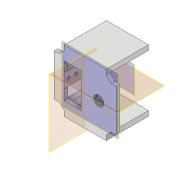
# Autodesk Inventor part: 30_Cube_Z_Focus_MGN_NEMA_base_v3
Saved by Autodesk Inventor 2022 (Build 260153000, 153)
## iProperties
Created: 2021-04-25
Part Number: 30_Cube_Z_Focus_MGN_NEMA_base_v3
Material: Generic
Document SubType Name: Modeling
Designer: diederichbenedict
Density: 1 g/cm^3
Appearance: Smooth - White
Author: diederichbenedict
Autodesk Inventor part; units mm, degrees
ref_plane "Work Plane1" through (0, 0, 6.7734) normal (0, 0, -1) x (-1, 0, 0)
sketch "Sketch1" plane through (0, 0, 6.7734) normal (0, 0, -1) x (-1, 0, 0)
  arc A0 (24.85, 22.85) -> (22.85, 24.85) centre (22.85, 22.85) ccw construction
  line L0 (22.85, 24.85) -> (-16.97, 24.85) construction
  line L1 (-16.97, 24.85) -> (-16.97, 21.15) construction
  line L2 (-16.97, 21.15) -> (16.97, 21.15) construction
  line L3 (16.97, 16.97) -> (16.97, 21.15) construction
  line L4 (21.15, 16.97) -> (16.97, 16.97) construction
  line L5 (21.15, 16.97) -> (21.15, -16.97) construction
  line L6 (21.15, -16.97) -> (24.85, -16.97) construction
  line L7 (24.85, -16.97) -> (24.85, 22.85) construction
  line L8 (23.75, 23.25) -> (23.75, 18.15) construction
  arc A1 (23.25, 17.65) -> (23.75, 18.15) centre (23.25, 18.15) ccw construction
  line L9 (23.25, 17.65) -> (20.8937, 17.65) construction
  arc A2 (20.5239, 17.8134) -> (20.8937, 17.65) centre (20.8937, 18.15) ccw construction
  line L10 (20.5239, 17.8134) -> (17.7803, 20.8273) construction
  arc A3 (17.65, 21.1639) -> (17.7803, 20.8273) centre (18.15, 21.1639) ccw construction
  line L11 (17.65, 21.1639) -> (17.65, 23.25) construction
  arc A4 (18.15, 23.75) -> (17.65, 23.25) centre (18.15, 23.25) ccw construction
  line L12 (18.15, 23.75) -> (23.25, 23.75) construction
  arc A5 (23.75, 23.25) -> (23.25, 23.75) centre (23.25, 23.25) ccw construction
  arc A6 (-24.85, -22.85) -> (-22.85, -24.85) centre (-22.85, -22.85) ccw construction
  line L13 (-22.85, -24.85) -> (16.97, -24.85) construction
  line L14 (16.97, -24.85) -> (16.97, -21.15) construction
  line L15 (16.97, -21.15) -> (-16.97, -21.15) construction
  line L16 (-16.97, -16.97) -> (-16.97, -21.15) construction
  line L17 (-21.15, -16.97) -> (-16.97, -16.97) construction
  line L18 (-21.15, -16.97) -> (-21.15, 16.97) construction
  line L19 (-21.15, 16.97) -> (-24.85, 16.97) construction
  line L20 (-24.85, 16.97) -> (-24.85, -22.85) construction
  line L21 (-20.8273, -17.7803) -> (-17.8134, -20.5239) construction
  arc A7 (-17.65, -20.8937) -> (-17.8134, -20.5239) centre (-18.15, -20.8937) ccw construction
  line L22 (-17.65, -20.8937) -> (-17.65, -23.25) construction
  arc A8 (-18.15, -23.75) -> (-17.65, -23.25) centre (-18.15, -23.25) ccw construction
  line L23 (-18.15, -23.75) -> (-23.25, -23.75) construction
  arc A9 (-23.75, -23.25) -> (-23.25, -23.75) centre (-23.25, -23.25) ccw construction
  line L24 (-23.75, -23.25) -> (-23.75, -18.15) construction
  arc A10 (-23.25, -17.65) -> (-23.75, -18.15) centre (-23.25, -18.15) ccw construction
  line L25 (-23.25, -17.65) -> (-21.1639, -17.65) construction
  arc A11 (-20.8273, -17.7803) -> (-21.1639, -17.65) centre (-21.1639, -18.15) ccw construction
  arc A12 (-22.85, 24.85) -> (-24.85, 22.85) centre (-22.85, 22.85) ccw construction
  line L26 (-22.85, 24.85) -> (16.97, 24.85) construction
  line L27 (16.97, 24.85) -> (16.97, 21.15) construction
  line L28 (16.97, 21.15) -> (-16.97, 21.15) construction
  line L29 (-16.97, 16.97) -> (-16.97, 21.15) construction
  line L30 (-21.15, 16.97) -> (-16.97, 16.97) construction
  line L31 (-21.15, 16.97) -> (-21.15, -16.97) construction
  line L32 (-21.15, -16.97) -> (-24.85, -16.97) construction
  line L33 (-24.85, -16.97) -> (-24.85, 22.85) construction
  line L34 (-20.8273, 17.7803) -> (-17.8134, 20.5239) construction
  arc A13 (-17.8134, 20.5239) -> (-17.65, 20.8937) centre (-18.15, 20.8937) ccw construction
  line L35 (-17.65, 20.8937) -> (-17.65, 23.25) construction
  arc A14 (-17.65, 23.25) -> (-18.15, 23.75) centre (-18.15, 23.25) ccw construction
  line L36 (-18.15, 23.75) -> (-23.25, 23.75) construction
  arc A15 (-23.25, 23.75) -> (-23.75, 23.25) centre (-23.25, 23.25) ccw construction
  line L37 (-23.75, 23.25) -> (-23.75, 18.15) construction
  arc A16 (-23.75, 18.15) -> (-23.25, 17.65) centre (-23.25, 18.15) ccw construction
  line L38 (-23.25, 17.65) -> (-21.1639, 17.65) construction
  arc A17 (-21.1639, 17.65) -> (-20.8273, 17.7803) centre (-21.1639, 18.15) ccw construction
  arc A18 (22.85, -24.85) -> (24.85, -22.85) centre (22.85, -22.85) ccw construction
  line L39 (22.85, -24.85) -> (-16.97, -24.85) construction
  line L40 (-16.97, -24.85) -> (-16.97, -21.15) construction
  line L41 (-16.97, -21.15) -> (16.97, -21.15) construction
  line L42 (16.97, -16.97) -> (16.97, -21.15) construction
  line L43 (21.15, -16.97) -> (16.97, -16.97) construction
  line L44 (21.15, -16.97) -> (21.15, 16.97) construction
  line L45 (21.15, 16.97) -> (24.85, 16.97) construction
  line L46 (24.85, 16.97) -> (24.85, -22.85) construction
  line L47 (23.75, -23.25) -> (23.75, -18.15) construction
  arc A19 (23.75, -18.15) -> (23.25, -17.65) centre (23.25, -18.15) ccw construction
  line L48 (23.25, -17.65) -> (20.8937, -17.65) construction
  arc A20 (20.8937, -17.65) -> (20.5239, -17.8134) centre (20.8937, -18.15) ccw construction
  line L49 (20.5239, -17.8134) -> (17.7803, -20.8273) construction
  arc A21 (17.7803, -20.8273) -> (17.65, -21.1639) centre (18.15, -21.1639) ccw construction
  line L50 (17.65, -21.1639) -> (17.65, -23.25) construction
  arc A22 (17.65, -23.25) -> (18.15, -23.75) centre (18.15, -23.25) ccw construction
  line L51 (18.15, -23.75) -> (23.25, -23.75) construction
  arc A23 (23.25, -23.75) -> (23.75, -23.25) centre (23.25, -23.25) ccw construction
  line L52 (24.85, 16.87) -> (16.87, 16.87)
  line L53 (16.87, -16.87) -> (24.85, -16.87)
  line L54 (24.85, -16.87) -> (24.85, 16.87)
  line L55 (-16.87, 24.85) -> (16.87, 24.85)
  line L56 (16.87, 24.85) -> (16.87, 13.87)
  line L57 (16.87, 13.87) -> (-16.87, 13.87)
  line L58 (-16.87, 13.87) -> (-16.87, 24.85)
  line L59 (-16.87, 16.87) -> (-24.85, 16.87)
  line L60 (-24.85, 16.87) -> (-24.85, -16.87)
  line L61 (-24.85, -16.87) -> (-16.87, -16.87)
  line L62 (-16.87, -16.87) -> (-16.87, 16.87)
  line L63 (-16.87, -24.85) -> (16.87, -24.85)
  line L64 (16.87, -24.85) -> (16.87, -13.87)
  line L65 (16.87, -13.87) -> (-16.87, -13.87)
  line L66 (-16.87, -13.87) -> (-16.87, -24.85)
  arc A24 (12.6573, -5.8482) -> (12.7994, -6.05) centre (12.9383, -5.8013) ccw construction
  line L67 (12.7994, -6.05) -> (16.97, -6.05) construction
  line L68 (16.97, -6.05) -> (16.97, 6.05) construction
  line L69 (12.7994, 6.05) -> (16.97, 6.05) construction
  arc A25 (12.7994, 6.05) -> (12.6573, 5.8482) centre (12.9383, 5.8013) ccw construction
  arc A26 (12.2641, 5.5514) -> (12.6573, 5.8482) centre (11.7553, 6.6343) ccw construction
  arc A27 (12.2641, 5.5514) -> (12.1529, 5.425) centre (12.3846, 5.3332) ccw construction
  line L70 (12.1141, 4.928) -> (12.1529, 5.425) construction
  arc A28 (11.8955, 4.7) -> (12.1141, 4.928) centre (11.8656, 4.9475) ccw construction
  line L71 (11.4444, 4.7) -> (11.8955, 4.7) construction
  arc A29 (11.1961, 4.9275) -> (11.4444, 4.7) centre (11.4444, 4.9493) ccw construction
  line L72 (11.1642, 5.293) -> (11.1961, 4.9275) construction
  arc A30 (11.1642, 5.293) -> (11.0112, 5.5514) centre (10.9164, 5.3208) ccw construction
  arc A31 (10.4933, 5.8954) -> (11.0112, 5.5514) centre (11.4026, 6.7024) ccw construction
  arc A32 (10.4933, 5.8954) -> (10.27, 6.05) centre (10.2627, 5.8008) ccw construction
  line L73 (9.67, 6.05) -> (10.27, 6.05) construction
  line L74 (9.17, 5.55) -> (9.67, 6.05) construction
  line L75 (9.17, 5.55) -> (9.17, -5.55) construction
  line L76 (9.17, -5.55) -> (9.67, -6.05) construction
  line L77 (9.67, -6.05) -> (10.27, -6.05) construction
  arc A33 (10.27, -6.05) -> (10.4933, -5.8954) centre (10.2627, -5.8008) ccw construction
  arc A34 (11.0112, -5.5514) -> (10.4933, -5.8954) centre (11.4026, -6.7024) ccw construction
  arc A35 (11.0112, -5.5514) -> (11.1642, -5.293) centre (10.9164, -5.3208) ccw construction
  line L78 (11.1642, -5.293) -> (11.1961, -4.9275) construction
  arc A36 (11.4444, -4.7) -> (11.1961, -4.9275) centre (11.4444, -4.9493) ccw construction
  line L79 (11.4444, -4.7) -> (11.8955, -4.7) construction
  arc A37 (12.1141, -4.928) -> (11.8955, -4.7) centre (11.8656, -4.9475) ccw construction
  line L80 (12.1141, -4.928) -> (12.1529, -5.425) construction
  arc A38 (12.1529, -5.425) -> (12.2641, -5.5514) centre (12.3846, -5.3332) ccw construction
  arc A39 (12.6573, -5.8482) -> (12.2641, -5.5514) centre (11.7553, -6.6343) ccw construction
  circle A40 centre (-22.53, 11.5) radius 1.025 construction
  circle A41 centre (-22.53, -11.5) radius 1.025 construction
  line L81 (-11.03, -14.1) -> (-11.03, -12.75) construction
  arc A42 (-11.03, 12.75) -> (-11.03, -12.75) centre (-11.03, 0) ccw construction
  line L82 (-11.03, 12.75) -> (-11.03, 14.1) construction
  line L83 (-11.03, 14.1) -> (-22.53, 14.1) construction
  arc A43 (-22.53, 14.1) -> (-25.13, 11.5) centre (-22.53, 11.5) ccw construction
  line L84 (-25.13, 11.5) -> (-25.13, -11.5) construction
  arc A44 (-25.13, -11.5) -> (-22.53, -14.1) centre (-22.53, -11.5) ccw construction
  line L85 (-22.53, -14.1) -> (-11.03, -14.1) construction
  circle A45 centre (-11.03, 0) radius 12.75 construction
  circle A46 centre (0.47, 11.5) radius 1.025 construction
  circle A47 centre (0.47, -11.5) radius 1.025 construction
  circle A48 centre (-22.53, -11.5) radius 1.025 construction
  circle A49 centre (-22.53, 11.5) radius 1.025 construction
  line L86 (-22.53, -14.1) -> (0.47, -14.1) construction
  arc A50 (-25.13, -11.5) -> (-22.53, -14.1) centre (-22.53, -11.5) ccw construction
  line L87 (-25.13, 11.5) -> (-25.13, -11.5) construction
  arc A51 (-22.53, 14.1) -> (-25.13, 11.5) centre (-22.53, 11.5) ccw construction
  line L88 (0.47, 14.1) -> (-22.53, 14.1) construction
  arc A52 (3.07, 11.5) -> (0.47, 14.1) centre (0.47, 11.5) ccw construction
  line L89 (3.07, -11.5) -> (3.07, 11.5) construction
  arc A53 (0.47, -14.1) -> (3.07, -11.5) centre (0.47, -11.5) ccw construction
  line L90 (-16.87, 13.87) -> (3.07, 13.87)
  line L91 (3.07, 13.87) -> (3.07, -13.87)
  line L92 (3.07, -13.87) -> (-16.87, -13.87)
  line L93 (-16.87, -13.87) -> (-16.87, 13.87)
  circle A54 centre (-11.03, 0) radius 2.75 construction
  line L94 (-16.87, 7.9971) -> (-16.87, -7.9971)
  circle A55 centre (-11.03, 0) radius 4
  line L95 (16.87, 6.05) -> (16.97, 6.05)
  line L96 (16.97, 6.05) -> (16.97, -6.05)
  line L97 (16.97, -6.05) -> (16.87, -6.05)
  line L98 (16.87, -6.05) -> (16.87, -4.7)
  line L99 (16.87, 4.7) -> (16.87, 6.05)
  line L100 (16.87, 16.87) -> (16.87, 6.05)
  line L101 (16.87, -6.05) -> (16.87, -16.87)
  point P0 (0, 0)
  point P1 (16.87, 16.87)
  point P2 (3.07, 13.87)
  point P3 (-16.87, 13.87)
  point P4 (-16.87, -13.87)
  dimension "d1" = 0.1
  dimension "d2" = 0.1
  dimension "d3" = 0.1
  dimension "d4" = 0.1
  dimension "d5" = 0.1
  dimension "d6" = 3
  dimension "d7" = 3
  dimension "d110" = 8
  constraints: 54 end point, 14 parallel, 14 point on line, 7 perpendicular, 6 horizontal, 1 centre point, 1 collinear
  measures "d1" distance between parallel lines of L30 L59
  measures "d2" distance between parallel lines of L1 L58
  measures "d3" distance between parallel lines of L27 L56
  measures "d4" distance between parallel lines of L43 L53
  measures "d5" distance between parallel lines of L16 L66
  measures "d6" distance between parallel lines of L59 L57
  measures "d7" distance between parallel lines of L61 L65
  measures "d110" diameter of A55
extrude "Extrusion1" add sketch "Sketch1" along normal blind 3 contours L54 L53 L64 L101 L97 L96 L95 L100 L56 L52 | L56 L57 L58 L55 | L64 L63 L66 L62 L65 | L91 L65 L62 L57 | L58 L62 L61 L60 L59
chamfer "Chamfer1" distance 3.9 angle 45 4 edges at (-16.87, -16.87, 5.2734) (16.87, -16.87, 5.2734) (16.87, 16.87, 5.2734) (-16.87, 16.87, 5.2734)
sketch "Sketch2" plane through (0, 0, 3.7734) normal (0, 0, -1) x (-1, 0, 0)
  line L0 (3.07, 13.87) -> (16.87, 13.87) projected
  line L1 (16.87, -13.87) -> (3.07, -13.87) projected
  line L2 (-16.87, -20.77) -> (-16.87, -24.85) construction
  line L3 (-16.87, -24.85) -> (16.87, -24.85) construction
  line L4 (16.87, -6.05) -> (16.87, -13.87) projected
  line L5 (16.87, 20.77) -> (16.87, 24.85) construction
  line L6 (16.87, 24.85) -> (-16.87, 24.85) construction
  line L7 (-16.87, 24.85) -> (-16.87, 20.77) construction
  line L8 (-20.77, 16.87) -> (-16.87, 20.77) construction
  line L9 (-20.77, 16.87) -> (-24.85, 16.87) construction
  line L10 (-24.85, 16.87) -> (-24.85, -16.87) construction
  line L11 (-24.85, -16.87) -> (-20.77, -16.87) construction
  line L12 (-16.87, -20.77) -> (-20.77, -16.87) construction
  line L13 (-13.8689, -21.8489) -> (-13.8689, -19.5269)
  line L14 (-13.8689, -19.5269) -> (-19.5269, -13.8689)
  line L15 (-19.5269, -13.8689) -> (-21.8489, -13.8689)
  line L16 (-21.8489, 13.8689) -> (-19.5269, 13.8689)
  line L17 (-19.5269, 13.8689) -> (-13.8689, 19.5269)
  line L18 (-13.8689, 19.5269) -> (-13.8689, 21.8489)
  line L19 (-13.8689, 21.8489) -> (-13.8689, 24.85)
  line L20 (-21.8489, 13.8689) -> (-24.85, 13.8689)
  line L21 (-21.8489, -13.8689) -> (-24.85, -13.8689)
  line L22 (-13.8689, -21.8489) -> (-13.8689, -24.85)
  line L23 (-11.5469, -21.8489) -> (-13.8689, -21.8489)
  line L24 (-21.8489, -13.8689) -> (-21.8489, -11.5469)
  line L25 (-21.8489, 11.5469) -> (-21.8489, 13.8689)
  line L26 (-13.8689, 21.8489) -> (-11.5469, 21.8489)
  line L27 (3.07, -13.87) -> (3.07, 13.87) projected
  line L28 (16.87, 13.87) -> (16.87, 6.05) projected
  line L29 (16.87, 6.05) -> (16.97, 6.05) projected
  line L30 (16.97, 6.05) -> (16.97, -6.05) projected
  line L31 (16.97, -6.05) -> (16.87, -6.05) projected
  line L32 (20.77, -16.87) -> (24.85, -16.87) construction
  line L33 (24.85, -16.87) -> (24.85, 16.87) construction
  line L34 (24.85, 16.87) -> (20.77, 16.87) construction
  line L35 (16.87, 20.77) -> (20.77, 16.87) construction
  line L36 (16.87, -24.85) -> (16.87, -20.77) construction
  line L37 (20.77, -16.87) -> (16.87, -20.77) construction
  line L38 (-13.87, 21.85) -> (13.87, 21.85) construction
  line L39 (13.87, 21.85) -> (13.87, 19.5274) construction
  line L40 (13.87, 19.5274) -> (19.5274, 13.87) construction
  line L41 (19.5274, 13.87) -> (21.85, 13.87) construction
  line L42 (21.85, 13.87) -> (21.85, -13.87) construction
  line L43 (21.85, -13.87) -> (19.5274, -13.87) construction
  line L44 (19.5274, -13.87) -> (13.87, -19.5274) construction
  line L45 (13.87, -19.5274) -> (13.87, -21.85) construction
  line L46 (13.87, -21.85) -> (-13.87, -21.85) construction
  line L47 (-13.87, -21.85) -> (-13.87, -19.5274) construction
  line L48 (-13.87, -19.5274) -> (-19.5274, -13.87) construction
  line L49 (-19.5274, -13.87) -> (-21.85, -13.87) construction
  line L50 (-21.85, -13.87) -> (-21.85, 13.87) construction
  line L51 (-21.85, 13.87) -> (-19.5274, 13.87) construction
  line L52 (-19.5274, 13.87) -> (-13.87, 19.5274) construction
  line L53 (-13.87, 19.5274) -> (-13.87, 21.85) construction
  line L54 (16.87, 24.85) -> (-16.87, 24.85) projected
  line L55 (13.87, 24.85) -> (13.87, 19.5274)
  line L56 (13.87, 19.5274) -> (19.5274, 13.87)
  line L57 (19.5274, 13.87) -> (24.85, 13.87)
  line L58 (24.85, -16.87) -> (24.85, 16.87) projected
  line L59 (24.85, -13.87) -> (19.5274, -13.87)
  line L60 (19.5274, -13.87) -> (13.87, -19.5274)
  line L61 (-16.87, -24.85) -> (16.87, -24.85) projected
  line L62 (13.87, -24.85) -> (13.87, -19.5274)
  line L63 (16.87, 24.85) -> (-16.87, 24.85) projected
  line L64 (13.87, 24.85) -> (16.87, 24.85)
  line L65 (16.87, 24.85) -> (16.87, 20.77)
  line L66 (16.87, 20.77) -> (20.77, 16.87)
  line L67 (24.85, 16.87) -> (20.77, 16.87) projected
  line L68 (24.85, 16.87) -> (20.77, 16.87)
  line L69 (24.85, -16.87) -> (24.85, 16.87) projected
  line L70 (24.85, 16.87) -> (24.85, 13.87)
  line L71 (24.85, -13.87) -> (24.85, -16.87)
  line L72 (24.85, -16.87) -> (20.77, -16.87)
  line L73 (20.77, -16.87) -> (16.87, -20.77)
  line L74 (16.87, -24.85) -> (16.87, -20.77) projected
  line L75 (16.87, -24.85) -> (16.87, -20.77)
  line L76 (16.87, -20.77) -> (16.87, -24.85)
  line L77 (16.87, -24.85) -> (-16.87, -24.85) projected
  line L78 (13.87, -24.85) -> (16.87, -24.85)
  point P0 (0, 0)
  dimension "d115" = 3
  constraints: 94 end point, 16 point on line, 6 collinear, 5 perpendicular, 1 horizontal, 1 vertical, 19 other
  measures "d115" distance between parallel lines of L6 L38
ref_plane "Work Plane2" through (-16.97, -24.85, 34.1) normal (0, 0, -1) x (0, 1, 0)
extrude "Extrusion2" add sketch "Sketch2" along normal blind 31.5 contours L65 L66 L67 L58 L57 L56 L55 L54 | L72 L73 L74 L61 L62 L60 L59 L58
sketch "Sketch4" plane through (-24.85, -16.87, 6.7734) normal (-1, 0, 0) x (0, 0, 1)
  line L0 (37.9, 11.3739) -> (37.9, 18.453) construction
  line L1 (23.6194, 18.453) -> (37.9, 18.453) construction
  arc A0 (22.1806, 18.453) -> (23.6194, 18.453) centre (22.9, 16.8577) ccw construction
  line L2 (-1.3806, 18.453) -> (22.1806, 18.453) construction
  arc A1 (-2.8194, 18.453) -> (-1.3806, 18.453) centre (-2.1, 16.8577) ccw construction
  line L3 (-31.3806, 18.453) -> (-2.8194, 18.453) construction
  arc A2 (-32.8194, 18.453) -> (-31.3806, 18.453) centre (-32.1, 16.8577) ccw construction
  line L4 (-42.1, 18.453) -> (-32.8194, 18.453) construction
  line L5 (-42.1, 11.3739) -> (-42.1, 18.453) construction
  line L6 (-42.1, 11.3739) -> (37.9, 11.3739) construction
  line L7 (37.9, 19.2506) -> (37.9, 22.3415) construction
  line L8 (-42.1, 22.3415) -> (37.9, 22.3415) construction
  line L9 (-42.1, 19.2506) -> (-42.1, 22.3415) construction
  line L10 (-42.1, 19.2506) -> (37.9, 19.2506) construction
  line L11 (-3, 3) -> (-3, 30.74) construction
  line L12 (-34.1, 33.84) -> (-34.1, -5.98) construction
  line L13 (-3, 11.3739) -> (-34.1, 11.3739)
  line L14 (-34.1, 11.3739) -> (-34.1, 22.3415)
  line L15 (-34.1, 22.3415) -> (-3, 22.3415)
  line L16 (-3, 22.3415) -> (-3, 11.3739)
  line L17 (-34.1, 11.3739) -> (-32.1, 11.3739)
  line L18 (-32.1, 11.3739) -> (-32.1, 3.0011)
  line L19 (-32.1, 3.0011) -> (-34.1, 3.0011)
  line L20 (-34.1, 3.0011) -> (-34.1, 11.3739)
  line L21 (-34.1, 22.3415) -> (-32.1, 22.3415)
  line L22 (-32.1, 22.3415) -> (-32.1, 30.7389)
  line L23 (-32.1, 30.7389) -> (-34.1, 30.7389)
  line L24 (-34.1, 30.7389) -> (-34.1, 22.3415)
  point P0 (-6.7734, 16.87)
  point P1 (-3, 3.0011)
  point P2 (-3, 30.7389)
  point P3 (-3, 33.74)
  point P4 (-3, 31.418)
  point P5 (-3, 0)
  dimension "d24" = 2
  constraints: 24 end point, 6 parallel, 5 point on line, 3 horizontal, 3 perpendicular
  measures "d24" distance of L18.end L19.end
ref_plane "Work Plane3" through (16.97, -5.4961, -37.9) normal (1, 0, 0) x (0, 1, 0)
extrude "Extrusion4" add sketch "Sketch4" against normal blind 7.88 contours L13 L14 L15 L16
sketch "Sketch5" plane through (-24.85, -16.87, 6.7734) normal (-1, 0, 0) x (0, 0, 1)
  circle A0 centre (-32.1, 16.87) radius 1.4
  circle A1 centre (-3.4423, 16.87) radius 1.4
  line L0 (0, -7.98) -> (-34.5, -7.98) projected
  line L1 (0, 41.72) -> (-34.5, 41.72) projected
  line L2 (0, -7.98) -> (-34.5, -7.98) projected
  point P0 (-6.7734, 16.87)
  dimension "d25" = 2.8
  dimension "d26" = 2.8
  dimension "d86" = 49.7
  dimension "d87" = 24.85
  dimension "d88" = 0
  constraints: 2 centre point
  measures "d25" diameter of A0
  measures "d26" diameter of A1
  measures "d86" distance between parallel lines of L1 L2
  measures "d87" distance from line of A0.centre L1
  measures "d88" vertical distance of A1.centre A0.centre
extrude "Extrusion5" cut sketch "Sketch5" against normal blind 10
pattern_linear "Rectangular Pattern1" count 5 spacing 6.25 along (0, 0, -1) of "Extrusion5"
ref_plane "Work Plane4" through (-25.03, -12.97, -12) normal (0, 0, 1) x (1, 0, 0)
sketch "Sketch12" plane through (-24.85, -16.87, 6.7734) normal (-1, 0, 0) x (0, 0, 1)
  ellipse E0 centre (-17.053, 16.87) end of major axis (-32.053, 16.87) minor radius 10.6066 projected
  circle A0 centre (-32.1, 16.87) radius 1.4 projected
  circle A1 centre (-22.1923, 16.87) radius 1.4 projected
  circle A2 centre (-15.9423, 16.87) radius 1.4 projected
  circle A3 centre (-9.6923, 16.87) radius 1.4 projected
  circle A4 centre (-3.4423, 16.87) radius 1.4 projected
  circle A5 centre (-28.4423, 16.87) radius 1.4 projected
  point P0 (-6.7734, 16.87)
  constraints: 1 other
hole "Hole2" at (-24.85, 0, -15.4189) at (-24.85, 0, -2.9189) at (-24.85, 0, 3.3311) at (-24.85, 0, -9.1689) at (-24.85, 0, -21.6689) direction (1, 0, 0) diameter 2.8 depth 8 tip angle 118 counterbore diameter 6 counterbore depth 3
ref_plane "Work Plane6" through (0, 0, -22) normal (0, 0, -1) x (-1, 0, 0)
ref_plane "Work Plane5" through (-16.97, -16.97, 0) normal (0, 0, 1) x (1, 0, 0)
ref_plane "Work Plane7" through (0, -16.87, 6.7734) normal (1, 0, 0) x (0, 0, -1)
ref_plane "Work Plane8" through (16.87, 0, 6.7734) normal (0, 1, 0) x (-1, 0, 0)
sketch "Skizze18" plane through (-24.85, -16.87, 6.7734) normal (-1, 0, 0) x (0, 0, 1)
  line L0 (0, 0) -> (-34.5, 0) projected
  line L1 (0, 0) -> (0, 33.74) projected
  line L2 (0, 33.74) -> (-34.5, 33.74) projected
  arc A0 (-31.2335, 15.7704) -> (-31.2335, 17.9696) centre (-28.4423, 16.87) ccw projected
  arc A1 (-31.2335, 17.9696) -> (-31.2335, 15.7704) centre (-32.1, 16.87) ccw projected
  circle A2 centre (-3.4423, 16.87) radius 3 projected
  circle A3 centre (-22.1923, 16.87) radius 3 projected
  circle A4 centre (-9.6923, 16.87) radius 3 projected
  circle A5 centre (-15.9423, 16.87) radius 3 projected
  line L3 (-3, 30.7389) -> (-34.5, 30.7389) projected
  line L4 (-34.1, 30.7389) -> (-3, 30.7389)
  line L5 (-3, 30.7389) -> (-3, 33.74)
  line L6 (-3, 33.74) -> (-34.1, 33.74)
  line L7 (-34.1, 33.74) -> (-34.1, 30.7389)
  line L8 (-3, 3.0011) -> (-34.5, 3.0011) projected
  line L9 (0, 0) -> (-34.5, 0) projected
  line L10 (-3, 3.0011) -> (-34.1, 3.0011)
  line L11 (-34.1, 3.0011) -> (-34.1, 0)
  line L12 (-34.1, 0) -> (-3, 0)
  line L13 (-3, 0) -> (-3, 3.0011)
  line L14 (-3, 22.3415) -> (-3, 30.74) projected
  line L15 (-34.1, 22.3415) -> (-3, 22.3415) projected
  line L16 (-34.1, 11.3739) -> (-34.1, 22.3415) projected
  line L17 (-3, 11.3739) -> (-34.1, 11.3739) projected
  line L18 (-3, 3) -> (-3, 11.3739) projected
  line L19 (-34.5, 30.74) -> (-34.5, 33.74) projected
  line L20 (-3, 30.74) -> (-34.5, 30.74) projected
  line L21 (-3, 3) -> (-34.5, 3) projected
  line L22 (-34.5, 0) -> (-34.5, 3) projected
  point P0 (-6.7734, 16.87)
  point P1 (-35.1, 0)
  point P2 (-34.1, 3.0011)
  point P3 (-3, 0)
  point P4 (-34.1, 0)
  constraints: 16 end point, 4 parallel, 3 point on line, 2 horizontal, 2 perpendicular
extrude "Extrusion14" cut sketch "Skizze18" against normal blind 10 contours L0 L11 L8 L13 | L5 L3 L7 L2
sketch "Skizze19" plane through (0, 0, 6.7734) normal (0, 0, 1) x (1, 0, 0)
  line L0 (-34.5437, 37.7032) -> (40.2308, 37.7032)
  line L1 (40.2308, 37.7032) -> (40.2308, -45.0753)
  line L2 (40.2308, -45.0753) -> (-34.5437, -45.0753)
  line L3 (-34.5437, -45.0753) -> (-34.5437, 37.7032)
  point P0 (0, 0)
  constraints: 8 end point, 2 parallel, 1 horizontal, 1 perpendicular
extrude "Extrusion15" cut sketch "Skizze19" against normal blind 34 keep common part
sketch "Skizze20" plane through (0, 0, 6.7734) normal (0, 0, 1) x (1, 0, 0)
  line L0 (-16.87, 24.85) -> (16.87, 24.85) projected
  line L1 (-16.87, -24.85) -> (16.87, -24.85) projected
  line L2 (16.87, 24.85) -> (16.87, 20.77) projected
  line L3 (-16.87, 24.85) -> (16.87, 24.85)
  line L4 (16.87, 24.85) -> (16.87, 20.85)
  line L5 (16.87, 20.85) -> (-16.87, 20.85)
  line L6 (-16.87, 20.85) -> (-16.87, 24.85)
  line L7 (-16.87, -13.87) -> (-16.87, -13.87) projected
  line L8 (-16.87, -24.85) -> (16.87, -24.85)
  line L9 (16.87, -24.85) -> (16.87, -20.85)
  line L10 (16.87, -20.85) -> (-16.87, -20.85)
  line L11 (-16.87, -20.85) -> (-16.87, -24.85)
  point P0 (0, 0)
  point P1 (-16.87, -20.77)
  point P2 (16.87, -24.85)
  point P3 (-16.87, -20.85)
  dimension "d104" = 4
  dimension "d105" = 4
  constraints: 16 end point, 4 parallel, 2 horizontal, 2 perpendicular, 2 point on line, 1 other
  measures "d104" distance of L3.end L4.end
  measures "d105" distance of L9.end L8.end
extrude "Extrusion16" add sketch "Skizze20" against normal blind 34
sketch "Skizze21" plane through (0, 0, -27.2266) normal (0, 0, -1) x (-1, 0, 0)
  line L0 (24.85, -5.4961) -> (24.85, 5.4715) projected
  line L1 (-16.87, -20.77) -> (-16.87, -24.85) projected
  line L2 (-16.87, -24.85) -> (-13.8689, -24.85) projected
  line L3 (-16.87, 24.85) -> (-16.87, 20.77) projected
  line L4 (16.87, 20.85) -> (16.87, 24.85) projected
  line L5 (16.87, 24.85) -> (-16.87, 24.85) projected
  line L6 (16.97, -5.4961) -> (24.85, -5.4961) projected
  line L7 (20.77, -16.87) -> (16.5258, -16.87) projected
  line L8 (24.85, -5.4961) -> (16.87, -5.4961)
  line L9 (16.87, -5.4961) -> (16.87, -16.87)
  line L10 (16.87, -16.87) -> (24.85, -16.87)
  line L11 (24.85, -16.87) -> (24.85, -5.4961)
  line L12 (24.85, -5.4961) -> (24.85, 5.4715) projected
  line L13 (16.5258, 16.87) -> (20.77, 16.87) projected
  line L14 (24.85, 5.4715) -> (16.87, 5.4715)
  line L15 (16.87, 5.4715) -> (16.87, 16.87)
  line L16 (16.87, 16.87) -> (24.85, 16.87)
  line L17 (24.85, 16.87) -> (24.85, 5.4715)
  line L18 (16.97, 5.4715) -> (16.97, -5.4961) projected
  line L19 (-16.87, 20.77) -> (-20.77, 16.87) projected
  line L20 (-20.77, 16.87) -> (-24.85, 16.87) projected
  line L21 (-24.85, 16.87) -> (-24.85, 13.8689) projected
  line L22 (-24.85, -16.87) -> (-20.77, -16.87) projected
  line L23 (-20.77, -16.87) -> (-16.87, -20.77) projected
  line L24 (-16.87, -20.77) -> (-16.87, -24.85) projected
  line L25 (-16.87, -24.85) -> (-13.8689, -24.85) projected
  line L26 (20.5128, -17.1272) -> (20.77, -16.87) projected
  line L27 (20.77, -16.87) -> (20.6183, -16.87) projected
  line L28 (-16.87, 24.85) -> (-16.87, 20.77) projected
  line L29 (-16.87, 20.77) -> (-20.77, 16.87) projected
  line L30 (-20.77, 16.87) -> (-24.85, 16.87) projected
  line L31 (-24.85, 16.87) -> (-24.85, 13.8689) projected
  line L32 (-24.85, -16.87) -> (-20.77, -16.87) projected
  line L33 (-20.77, -16.87) -> (-16.87, -20.77) projected
  line L34 (20.5128, -17.1272) -> (20.77, -16.87) projected
  line L35 (20.77, -16.87) -> (20.6183, -16.87) projected
  line L36 (16.87, 20.85) -> (16.87, 24.85) projected
  line L37 (16.87, 24.85) -> (-16.87, 24.85) projected
  line L38 (20.6183, -16.87) -> (20.5128, -17.1272) projected
  line L39 (-24.85, 13.8689) -> (-19.5269, 13.8689) projected
  line L40 (-19.5269, 13.8689) -> (-13.8689, 19.5269) projected
  line L41 (-13.8689, 19.5269) -> (-13.8689, 20.85) projected
  line L42 (-13.8689, 20.85) -> (16.87, 20.85) projected
  line L43 (-13.8689, -24.85) -> (-13.8689, -19.5269) projected
  line L44 (-13.8689, -19.5269) -> (-19.5269, -13.8689) projected
  line L45 (-19.5269, -13.8689) -> (-24.85, -13.8689) projected
  line L46 (-24.85, -13.8689) -> (-24.85, -16.87) projected
  line L47 (20.6183, -16.87) -> (20.5128, -17.1272) projected
  line L48 (-24.85, 13.8689) -> (-19.5269, 13.8689) projected
  line L49 (-19.5269, 13.8689) -> (-13.8689, 19.5269) projected
  line L50 (-13.8689, 19.5269) -> (-13.8689, 20.85) projected
  line L51 (-13.8689, 20.85) -> (16.87, 20.85) projected
  line L52 (-13.8689, -24.85) -> (-13.8689, -19.5269) projected
  line L53 (-13.8689, -19.5269) -> (-19.5269, -13.8689) projected
  line L54 (-19.5269, -13.8689) -> (-24.85, -13.8689) projected
  line L55 (-24.85, -13.8689) -> (-24.85, -16.87) projected
  line L56 (24.85, 5.4715) -> (16.97, 5.4715) projected
  line L57 (16.97, -5.4961) -> (24.85, -5.4961) projected
  point P0 (0, 0)
  point P1 (-16.97, -5.4961)
  point P2 (24.85, 13.8689)
  point P3 (24.85, -13.8689)
  constraints: 16 end point, 4 parallel, 2 horizontal, 2 perpendicular, 2 point on line
extrude "Extrusion17" add sketch "Skizze21" against normal blind 2 contours L11 L10 L7 L9 L8 L6 | L14 L15 L13 L16 L17
sketch "Skizze22" plane through (0, 0, 3.7734) normal (0, 0, -1) x (-1, 0, 0)
  circle A0 centre (-11.3313, 0) radius 3.075 projected
  circle A1 centre (-11.3313, 0) radius 1.5
  circle A2 centre (-11.3313, 0) radius 2.5
  point P0 (0, 0)
  dimension "d111" = 3
  dimension "d112" = 5
  constraints: 2 centre point, 2 coincident
  measures "d111" diameter of A1
  measures "d112" diameter of A2
extrude "Extrusion18" add sketch "Skizze22" against normal blind 3 draft -2 contours A2
equation "\"d2\" = d1"
equation "\"d3\" = d1"
equation "\"d4\" = d1"
equation "\"d5\" = d1"
body "Solid1"
